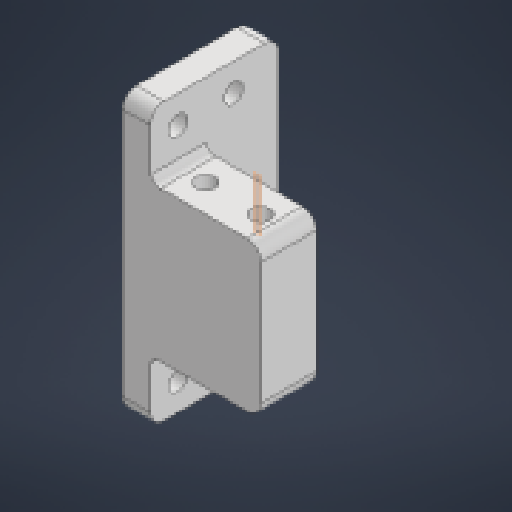
# Autodesk Inventor part: HardStop
Saved by Autodesk Inventor 2026.1 (Build 301233000, 233)
## iProperties
Created: 2025-09-08
Part Number: HardStop
Material: Generic
Document SubType Name: Modeling
Designer: Teddy
Density: 1 g/cm^3
Appearance: Default
Author: Teddy
Autodesk Inventor part; units mm, degrees
ref_plane "YZ Plane" through (0, 0, 0) normal (1, 0, 0) x (0, 1, 0)
ref_plane "XZ Plane" through (0, 0, 0) normal (0, 1, 0) x (-1, 0, 0)
ref_plane "XY Plane" through (0, 0, 0) normal (0, 0, 1) x (1, 0, 0)
ref_plane "Work Plane1" through (22.225, 0, 0) normal (0, 0, 1) x (1, 0, 0)
sketch "Sketch1" plane through (22.225, 0, 0) normal (0, 0, 1) x (1, 0, 0)
  line L0 (-23.8125, 10.8902) -> (-23.8125, 0) projected
  line L1 (-23.8125, -39.6875) -> (-23.8125, -50.5778) projected
  line L2 (-23.8125, 11.9062) -> (-35.2425, 11.9062)
  line L3 (-35.2425, 11.9062) -> (-35.2425, -51.5938)
  line L4 (-35.2425, -51.5938) -> (-23.8125, -51.5938)
  line L5 (-23.8125, -51.5938) -> (-23.8125, 11.9062)
  line L6 (-23.8125, -51.5938) -> (-22.225, -51.5938) projected
  line L7 (-22.225, 11.9062) -> (-23.8125, 11.9062) projected
  line L8 (-23.8125, 11.9062) -> (-23.8125, 18.2562)
  line L9 (-23.8125, 18.2562) -> (-35.2425, 18.2562)
  line L10 (-35.2425, 18.2562) -> (-35.2425, 11.9062)
  point P0 (-22.225, 0)
  point P1 (-23.8125, -50.5778)
  point P2 (-23.8125, 0)
  dimension "d0" = 11.43
  dimension "d14" = 6.35
  constraints: 14 end point, 3 perpendicular, 2 coincident, 2 parallel, 1 horizontal, 1 horizontal alignment, 1 point on line
  measures "d0" distance between parallel lines of L5 L3
  measures "d14" distance between parallel lines of L9 L2
ref_plane "Work Plane2" through (-1.5875, 3.7528, -29.4386) normal (0, 0, -1) x (0, 1, 0)
extrude "Extrusion1" add sketch "Sketch1" against normal up to surface (29.4386 mm away)
sketch "Sketch2" plane through (-13.0175, -51.5938, 0) normal (-1, 0, 0) x (0, 0, 1)
  circle A0 centre (-6.35, 57.15) radius 2.1844 projected
  circle A1 centre (-19.05, 57.15) radius 2.1844 projected
  circle A2 centre (-19.05, 6.35) radius 2.1844 projected
  circle A3 centre (-6.35, 6.35) radius 2.1844 projected
  point P0 (0, 51.5938)
extrude "Extrusion2" cut sketch "Sketch2" against normal blind 25.4
fillet "Fillet1" radius 3.175 4 edges at (-7.3025, -51.5938, -29.4386) (-7.3025, -51.5938, 0) (-7.3025, 18.2562, 0) (-7.3025, 18.2563, -29.4386)
sketch "Sketch3" plane through (22.225, 0, 0) normal (0, 0, 1) x (1, 0, 0)
  arc A0 (-21.4313, -37.3063) -> (-23.8125, -39.6875) centre (-21.4313, -39.6875) ccw projected
  line L0 (-21.4313, -37.3063) -> (-0.7937, -37.3063) projected
  arc A1 (-23.8125, 0) -> (-21.4313, -2.3813) centre (-21.4313, 0) ccw projected
  line L1 (-13.4239, -2.3813) -> (-21.4313, -2.3813) projected
  line L2 (-23.8125, -48.4188) -> (-23.8125, 8.7312) projected
  line L3 (1.5875, -50.5778) -> (1.5875, -39.6875) projected
  line L4 (1.5875, -39.6875) -> (1.5875, 1.6693)
  line L5 (-0.7937, -37.3063) -> (1.5875, -37.3063)
  line L6 (-13.4239, -2.3813) -> (1.5875, -2.3813)
  line L7 (1.5875, -37.0523) -> (-0.7937, -37.0523)
  line L8 (-0.7937, -37.0523) -> (-21.4313, -37.0523)
  arc A2 (-21.4313, -37.0523) -> (-24.0665, -39.6875) centre (-21.4313, -39.6875) ccw
  arc A3 (-24.0665, 0) -> (-21.4313, -2.6353) centre (-21.4313, 0) ccw
  line L9 (-21.4313, -2.6353) -> (-13.4239, -2.6353)
  line L10 (-13.4239, -2.6353) -> (1.5875, -2.6353)
  point P0 (-22.225, 0)
  point P1 (1.5875, -37.0523)
  point P2 (1.5875, -2.6353)
  point P3 (-23.8125, -1.1288)
  point P4 (-23.8125, -38.5587)
  dimension "d6" = 0.254
  dimension "d7" = 0.254
  constraints: 14 end point, 4 point on circle, 2 centre point, 2 perpendicular, 2 point on line, 1 vertical, 4 other
  measures "d6" distance between parallel lines of L0 L8
  measures "d7" distance between parallel lines of L1 L9
extrude "Extrusion3" add sketch "Sketch3" against normal blind 12.7 contours L2 A3 L9 L10 L4 L7 L8 A2
fillet "Fillet2" radius 3.175 2 edges at (23.8125, -37.0523, -6.35) (23.8125, -2.6352, -6.35)
sketch "Sketch4" plane through (0.7937, -37.0523, -12.7) normal (0, -1, 0) x (1, 0, 0)
  circle A0 centre (3.9688, 6.35) radius 2.1844 projected
  circle A1 centre (16.6688, 6.35) radius 2.1844 projected
  point P0 (-0.7937, 12.7)
extrude "Extrusion4" cut sketch "Sketch4" against normal up to surface (34.417 mm away)
fillet "Fillet3" radius 3.175 1 edges at (-13.0175, -51.5938, -14.7193)
body "Solid1"
